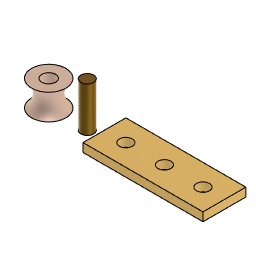
ExoArm v0 (Autodesk Fusion 360 design; units mm, degrees)
Autodesk Fusion 360 part; units mm, degrees
note: some values were not read from the file. Chosen so that the rebuilt part matches the saved one: which bodies a step acts on; which face or edge a step refers to.
sketch "Sketch1" plane through (0, 0, 0) normal (0, 0, 1) x (1, 0, 0)
  circle A0 centre (0, 0) radius 20
  circle A1 centre (0, 0) radius 8
  line L0 (0, 0) -> (20, 0)
  line L1 (20, 0) -> (8, 0)
  line L2 (8, 0, 0) -> (8, 0, 30)
  line L3 (8, 0) -> (13, 0)
  line L4 (13, 0, 0) -> (13, 0, 30)
  line L5 (13, 0, 30) -> (20, 0, 30)
  arc A2 through (20, 0, 30) (13, 0, 15) (20, 0, 0)
  line L6 (8, 0, 30) -> (20, 0, 30)
  dimension "d1" = 40
  dimension "d2" = 16
  dimension "d3" = 30
  dimension "d4" = 5
  dimension "d5" = 30
  dimension "d6" = 7
  constraint coincident A0.centre A1.centre
  constraint concentric A0 A1
  constraint coincident A0 L0.end
  constraint horizontal L0
  constraint coincident A1 L1.end
  constraint coincident L0 L1.end
  measures "d1" diameter of A0
  measures "d2" diameter of A1
  measures "d3" distance of L1.end L3.start
  measures "d4" distance of L1.end L3.end
  measures "d6" distance of L3.end L0.end
sketch "Sketch1 (curves on the plane with normal 0, 1, 0 at 0 mm)" plane through (0, 0, 0) normal (0, 1, 0) x (-1, 0, 0)
  line L0 (0, 0) -> (-20, 0)
  line L1 (-20, 0) -> (-8, 0)
  line L2 (-8, 0) -> (-8, 30)
  line L3 (-8, 0) -> (-13, 0)
  line L4 (-13, 0) -> (-13, 30)
  line L5 (-13, 30) -> (-20, 30)
  arc A0 (-20, 30) -> (-20, 0) centre (-32.5714, 15) cw
  line L6 (-8, 30) -> (-20, 30)
sweep "Sweep1" add profiles "Sketch1 (curves on the plane with normal 0, 1, 0 at 0 mm)" path "Sketch1" along A1 section 1 makes body 1
sketch "Sketch2" plane through (0, 0, 0) normal (0, 0, 1) x (1, 0, 0)
  line L0 (61.2298, 22.7494) -> (201.2298, 22.7494)
  line L1 (201.2298, 22.7494) -> (201.2298, -27.2506)
  line L2 (201.2298, -27.2506) -> (61.2298, -27.2506)
  line L3 (61.2298, -27.2506) -> (61.2298, 22.7494)
  circle A0 centre (86.2298, -2.2506) radius 7.5
  circle A1 centre (131.2298, -2.2506) radius 7.5
  circle A2 centre (176.2298, -2.2506) radius 7.5
  dimension "d13" = 140
  dimension "d14" = 50
  dimension "d16" = 45
  dimension "d17" = 15
  dimension "d18" = 15
  dimension "d19" = 15
  constraint horizontal L0
  constraint vertical L1
  constraint horizontal L2
  constraint vertical L3
  measures "d13" distance of L0.start L0.end
  measures "d14" distance of L0.start L2.end
  measures "d16" distance of A0.centre A1.centre
  measures "d17" diameter of A0
  measures "d18" diameter of A1
  measures "d19" diameter of A2
move_body "Move1" bodies 1 to x (1, 0, 0) y (0, 1, 0) z (0, 0, 1) at (86.2298, -2.2506, 0)
extrude "Extrude1" add sketch "Sketch2" along normal blind 32 separate body contours A0 | A1 | A2 makes body 2 at (93.7205, -2.6244, 21.3333) makes body 3 at (138.7205, -2.6244, 21.3333) makes body 4 at (183.7205, -2.6244, 21.3333)
extrude "Extrude2" add sketch "Sketch2" against normal blind 10 contours L0 L1 L2 L3 | A0 | A1 | A2 bodies 2 3 4
sketch "Sketch3" plane through (0, 0, 32) normal (0, 0, 1) x (-1, 0, 0)
  circle A0 centre (-86.2298, 2.2506) radius 7.5
  line L0 (-61.2298, -22.7494) -> (-201.2298, -22.7494)
  line L1 (-201.2298, -22.7494) -> (-201.2298, 27.2506)
  line L2 (-201.2298, 27.2506) -> (-61.2298, 27.2506)
  line L3 (-61.2298, 27.2506) -> (-61.2298, -22.7494)
  dimension "d26" = 140
  dimension "d27" = 50
  constraint horizontal L0
  constraint vertical L1
  constraint horizontal L2
  constraint vertical L3
  measures "d26" distance of L0.start L0.end
  measures "d27" distance of L0.start L2.end
extrude "Extrude3" add sketch "Sketch3" along normal blind 10 contours A0 | L0 L1 L2 L3 bodies 2
split "Split1" by plane through (0, 0, 32) normal (0, 0, -1) bodies 2 makes body 5 at (107.8964, 6.0827, -10)
split "Split2" by plane through (0, 0, 0) normal (0, 0, 1) bodies 5 makes body 6 at (138.7205, -2.6244, 21.3333) makes body 7 at (93.7205, -2.6244, 21.3333) makes body 8 at (183.7205, -2.6244, 21.3333)
delete_body "RemoveBody1" bodies 6
delete_body "RemoveBody2" bodies 7
delete_body "RemoveBody3" bodies 2
move_body "Move5" bodies 8 to x (1, 0, 0) y (0, 1, 0) z (0, 0, 1) at (-135, 0, 0)
extrude "Extrude4" add 1 faces at (39.9798, -2.9419, 32) along direction (0, 0, 1) blind 10 on bodies 8 bodies 8
extrude "Extrude5" add 1 faces at (39.9798, -2.9419, 0) along direction (0, 0, -1) blind 10 on bodies 8 bodies 8
extrude "Extrude6" cut sketch "Sketch2" against normal blind 40 contours A0 | A1 | A2 bodies 5
move_body "Move6" bodies 1 to x (1, 0, 0) y (0, 1, 0) z (0, 0, 1) at (-90, 0, -10)
